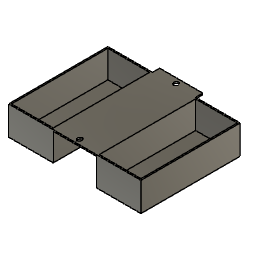
Load basket version 1 v3 (Autodesk Fusion 360 design; units mm, degrees)
Autodesk Fusion 360 part; units mm, degrees
note: some values were not read from the file. Set by a fixed rule: which face or edge a step refers to.
sketch "Sketch1" plane through (0, 0, 350) normal (0, 0, 1) x (-1, 0, 0)
  line L0 (-26.0008, 95.0009) -> (-26.0008, -144.9991)
  line L1 (-26.0008, -144.9991) -> (23.9992, -144.9991)
  line L2 (23.9992, -144.9991) -> (23.9992, 95.0009)
  line L3 (23.9992, 95.0009) -> (-26.0008, 95.0009)
  circle A0 centre (-0.9844, 75.5009) radius 10
  circle A1 centre (-1.0008, 8.5009) radius 10
  circle A2 centre (-1.0008, -58.4991) radius 10
  circle A3 centre (-0.9479, -125.4989) radius 10
  line L4 (5.9992, -44.9991) -> (5.9992, -4.9991)
  arc A4 (15.9992, -4.9991) -> (5.9992, -4.9991) centre (10.9992, -4.9991) ccw
  line L5 (15.9992, -4.9991) -> (15.9992, -44.9991)
  arc A5 (5.9992, -44.9991) -> (15.9992, -44.9991) centre (10.9992, -44.9991) ccw
  line L6 (-18.0008, 25.0009) -> (-18.0008, 60.0009)
  arc A6 (-8.0008, 60.0009) -> (-18.0008, 60.0009) centre (-13.0008, 60.0009) ccw
  line L7 (-8.0008, 60.0009) -> (-8.0008, 25.0009)
  arc A7 (-18.0008, 25.0009) -> (-8.0008, 25.0009) centre (-13.0008, 25.0009) ccw
  circle A8 centre (-0.9844, 42.0009) radius 4
  line L8 (-8.0008, -74.9991) -> (-8.0013, -109.9281)
  arc A9 (-18.0003, -109.9281) -> (-8.0013, -109.9281) centre (-13.0008, -109.9991) ccw
  line L9 (-18.0003, -109.9281) -> (-18.0008, -74.9991)
  arc A10 (-8.0008, -74.9991) -> (-18.0008, -74.9991) centre (-13.0008, -74.9991) ccw
  circle A11 centre (-0.9479, -91.9989) radius 4
  circle A12 centre (-1.0008, -24.9991) radius 4
  line L10 (-8.0008, -4.9991) -> (-8.0008, -44.9991)
  arc A13 (-18.0008, -44.9991) -> (-8.0008, -44.9991) centre (-13.0008, -44.9991) ccw
  line L11 (-18.0008, -44.9991) -> (-18.0008, -4.9991)
  arc A14 (-8.0008, -4.9991) -> (-18.0008, -4.9991) centre (-13.0008, -4.9991) ccw
  line L12 (5.9992, 25.0009) -> (5.9992, 60.0009)
  arc A15 (15.9992, 60.0009) -> (5.9992, 60.0009) centre (10.9992, 60.0009) ccw
  line L13 (15.9992, 60.0009) -> (15.9992, 25.0009)
  arc A16 (5.9992, 25.0009) -> (15.9992, 25.0009) centre (10.9992, 25.0009) ccw
  line L14 (5.9992, -109.9991) -> (5.9992, -74.9991)
  arc A17 (15.9992, -74.9991) -> (5.9992, -74.9991) centre (10.9992, -74.9991) ccw
  line L15 (15.9992, -74.9991) -> (15.9992, -109.9991)
  arc A18 (5.9992, -109.9991) -> (15.9992, -109.9991) centre (10.9992, -109.9991) ccw
  circle A19 centre (-0.9844, 42.0009) radius 4
  line L16 (26, 45) -> (26, 35)
  line L17 (26, 35) -> (-28, 35)
  line L18 (-28, 35) -> (-28, 45)
  line L19 (-28, 45) -> (-28, 49)
  line L20 (-28, 49) -> (26, 49)
  line L21 (26, 49) -> (26, 45)
  circle A20 centre (-0.9479, -91.9989) radius 4
  line L22 (-1, -85) -> (26, -85)
  line L23 (26, -85) -> (26, -98)
  line L24 (26, -98) -> (26, -99)
  line L25 (26, -99) -> (-28, -99)
  line L26 (-28, -99) -> (-28, -86)
  line L27 (-28, -86) -> (-28, -85)
  line L28 (-28, -85) -> (-1, -85)
  constraint concentric A8 A19
  constraint vertical L16
  constraint horizontal L17
  constraint vertical L18
  constraint vertical L19
  constraint horizontal L20
  constraint vertical L21
  constraint concentric A11 A20
  constraint perpendicular L2 L22
  constraint perpendicular L22 L23
  constraint parallel L2 L24
  constraint perpendicular L0 L25
  constraint perpendicular L25 L26
  constraint perpendicular L22 L27
  constraint parallel L22 L28
extrude "Extrude1" add sketch "Sketch1" along normal blind 2 contours L0 L9 L25 L28 | L0 L25 L26 L27 L28 | L8 L9 L25 L28 | L2 L22 L23 L24 L25 | L2 L15 L22 L25 | L8 L14 L22 L25 L28 | L14 L15 L22 L25 makes body 1
extrude "Extrude2" add sketch "Sketch1" along normal blind 2 separate body contours L0 L6 L17 L20 | L0 L17 L18 L19 L20 | L6 L7 L17 L20 | L2 L16 L17 L20 L21 | L2 L13 L17 L20 | L7 L12 L17 L20 | L12 L13 L17 L20 makes body 2
extrude "Extrude3" add 4 faces at (28, -46.3333, 350.6667) (28, -38.3333, 350.6667) (28, 85.6667, 350.6667) (28, 94.6667, 350.6667) along direction (1, 0, 0) blind 2 on bodies 1 2 bodies 2 1
sketch "Sketch3" plane through (30, 0, 0) normal (1, 0, 0) x (0, 1, 0)
  line L0 (-49, 350) -> (-35, 350)
  line L1 (-35, 350) -> (-35, 352)
  line L2 (-35, 352) -> (-49, 352)
  line L3 (-49, 352) -> (-49, 350)
  line L4 (-49, 352) -> (-35, 352)
  line L5 (-35, 352) -> (-35, 312)
  line L6 (-35, 312) -> (-49, 312)
  line L7 (-49, 312) -> (-49, 352)
  line L8 (85.0431, 352) -> (99, 352)
  line L9 (99, 352) -> (99, 312)
  line L10 (99, 312) -> (85.0431, 312)
  line L11 (85.0431, 352) -> (84.9998, 352)
  line L12 (84.9998, 352) -> (84.9998, 312)
  line L13 (84.9998, 312) -> (85.0431, 312)
  constraint horizontal L4
  constraint vertical L5
  constraint horizontal L6
  constraint vertical L7
  constraint coincident L2.end L3.start
  constraint horizontal L8
  constraint vertical L9
  constraint horizontal L10
  constraint horizontal L11
  constraint vertical L12
  constraint horizontal L13
extrude "Extrude4" add sketch "Sketch3" along normal blind 2 bodies 1 2
extrude "Extrude5" add 1 faces at (12, -35, 351.3333) along direction (0, 1, 0) blind 125 on bodies 2 bodies 2 1
extrude "Extrude6" cut sketch "Sketch1" along normal blind 15 contours A8 A19 | A11 A20 bodies 2
sketch "Sketch4" plane through (32, 0, 0) normal (1, 0, 0) x (0, 1, 0)
  line L0 (-49, 312) -> (99, 312)
  line L1 (99, 312) -> (99, 352)
  line L2 (99, 352) -> (-49, 352)
  line L3 (-49, 352) -> (-49, 312)
  line L4 (-49, 352) -> (-47, 352)
  line L5 (-47, 352) -> (-47, 312)
  line L6 (-47, 312) -> (-49, 312)
  line L7 (-49, 312) -> (-49, 352)
  line L8 (-47, 314) -> (99, 314)
  line L9 (99, 314) -> (99, 312)
  line L10 (99, 312) -> (-47, 312)
  line L11 (-47, 312) -> (-47, 314)
  line L12 (97, 314) -> (99, 314)
  line L13 (99, 314) -> (99, 352)
  line L14 (99, 352) -> (97, 352)
  line L15 (97, 352) -> (97, 314)
  constraint horizontal L4
  constraint vertical L5
  constraint horizontal L6
  constraint vertical L7
  constraint coincident L2.end L3.start
  constraint horizontal L8
  constraint vertical L9
  constraint horizontal L10
  constraint vertical L11
  constraint coincident L0.end L1.start
  constraint coincident L5 L8.start
  constraint horizontal L12
  constraint vertical L13
  constraint horizontal L14
  constraint vertical L15
  constraint coincident L1.end L2.start
  constraint coincident L8 L12.start
extrude "Extrude7" add sketch "Sketch4" along normal blind 30 contours L0 L2 L3 L4 L5 L6 L7 L11 | L0 L1 L5 L8 L9 L10 L11 L12 | L1 L2 L8 L12 L13 L14 L15 bodies 2
sketch "Sketch5" plane through (0, 0, 314) normal (0, 0, 1) x (-1, 0, 0)
  line L0 (-32, -97) -> (-32, 47)
  line L1 (-32, 47) -> (-62, 47)
  line L2 (-62, 47) -> (-62, -97)
  line L3 (-62, -97) -> (-32, -97)
  line L4 (-60, 47) -> (-62, 47)
  line L5 (-62, 47) -> (-62, -97)
  line L6 (-62, -97) -> (-60, -97)
  line L7 (-60, -97) -> (-60, 47)
  constraint horizontal L4
  constraint vertical L5
  constraint horizontal L6
  constraint vertical L7
  constraint coincident L2.end L3.start
  constraint coincident L1 L4.start
extrude "Extrude8" add sketch "Sketch5" along normal blind 38 contours L1 L2 L3 L4 L5 L6 L7 bodies 2
sketch "Sketch6" plane through (62, 0, 0) normal (1, 0, 0) x (0, 1, 0)
  line L0 (99, 312) -> (99, 352)
  line L1 (99, 352) -> (97, 352)
  line L2 (97, 352) -> (-47, 352)
  line L3 (-49, 352) -> (-49, 312)
  line L4 (-49, 312) -> (99, 312)
  line L5 (-47, 352) -> (99, 312) construction
  line L6 (99, 352) -> (-49, 312) construction
  line L7 (24, 347) -> (26, 347)
  line L8 (26, 347) -> (26, 317)
  line L9 (26, 317) -> (24, 317)
  line L10 (24, 317) -> (24, 347)
  line L11 (31, 347) -> (33, 347)
  line L12 (33, 347) -> (33, 317)
  line L13 (33, 317) -> (31, 317)
  line L14 (31, 317) -> (31, 347)
  line L15 (38, 347) -> (40, 347)
  line L16 (40, 347) -> (40, 317)
  line L17 (40, 317) -> (38, 317)
  line L18 (38, 317) -> (38, 347)
  line L19 (45, 317) -> (47, 317)
  line L20 (47, 317) -> (47, 347)
  line L21 (47, 347) -> (45, 347)
  line L22 (45, 347) -> (45, 317)
  line L23 (52, 347) -> (54, 347)
  line L24 (54, 347) -> (54, 317)
  line L25 (54, 317) -> (52, 317)
  line L26 (52, 317) -> (52, 347)
  line L27 (59, 317) -> (61, 317)
  line L28 (61, 317) -> (61, 347)
  line L29 (61, 347) -> (59, 347)
  line L30 (59, 347) -> (59, 317)
  line L31 (66, 347) -> (68, 347)
  line L32 (68, 347) -> (68, 317)
  line L33 (68, 317) -> (66, 317)
  line L34 (66, 317) -> (66, 347)
  line L35 (73, 317) -> (75, 317)
  line L36 (75, 317) -> (75, 347)
  line L37 (75, 347) -> (73, 347)
  line L38 (73, 347) -> (73, 317)
  line L39 (80, 347) -> (82, 347)
  line L40 (82, 347) -> (82, 317)
  line L41 (82, 317) -> (80, 317)
  line L42 (80, 317) -> (80, 347)
  line L43 (87, 347) -> (89, 347)
  line L44 (89, 347) -> (89, 317)
  line L45 (89, 317) -> (87, 317)
  line L46 (87, 317) -> (87, 347)
  line L47 (94, 347) -> (96, 347)
  line L48 (96, 347) -> (96, 317)
  line L49 (96, 317) -> (94, 317)
  line L50 (94, 317) -> (94, 347)
  line L51 (19, 347) -> (17, 347)
  line L52 (17, 347) -> (17, 317)
  line L53 (17, 317) -> (19, 317)
  line L54 (19, 317) -> (19, 347)
  line L55 (12, 347) -> (10, 347)
  line L56 (10, 347) -> (10, 317)
  line L57 (10, 317) -> (12, 317)
  line L58 (12, 317) -> (12, 347)
  line L59 (5, 317) -> (3, 317)
  line L60 (3, 317) -> (3, 347)
  line L61 (3, 347) -> (5, 347)
  line L62 (5, 347) -> (5, 317)
  line L63 (-2, 347) -> (-4, 347)
  line L64 (-4, 347) -> (-4, 317)
  line L65 (-4, 317) -> (-2, 317)
  line L66 (-2, 317) -> (-2, 347)
  line L67 (-9, 317) -> (-11, 317)
  line L68 (-11, 317) -> (-11, 347)
  line L69 (-11, 347) -> (-9, 347)
  line L70 (-9, 347) -> (-9, 317)
  line L71 (-16, 347) -> (-18, 347)
  line L72 (-18, 347) -> (-18, 317)
  line L73 (-18, 317) -> (-16, 317)
  line L74 (-16, 317) -> (-16, 347)
  line L75 (-23, 317) -> (-25, 317)
  line L76 (-25, 317) -> (-25, 347)
  line L77 (-25, 347) -> (-23, 347)
  line L78 (-23, 347) -> (-23, 317)
  line L79 (-30, 317) -> (-32, 317)
  line L80 (-32, 317) -> (-32, 347)
  line L81 (-32, 347) -> (-30, 347)
  line L82 (-30, 347) -> (-30, 317)
  line L83 (-37, 347) -> (-39, 347)
  line L84 (-39, 347) -> (-39, 317)
  line L85 (-39, 317) -> (-37, 317)
  line L86 (-37, 317) -> (-37, 347)
  line L87 (-44, 347) -> (-46, 347)
  line L88 (-46, 347) -> (-46, 317)
  line L89 (-46, 317) -> (-44, 317)
  line L90 (-44, 317) -> (-44, 347)
  line L91 (-47, 352) -> (-49, 352)
  constraint coincident L2.end L5.start
  constraint coincident L0.start L4.end
  constraint coincident L0.end L1.start
  constraint coincident L3.end L4.start
  constraint horizontal L7
  constraint vertical L8
  constraint horizontal L9
  constraint vertical L10
  constraint horizontal L11
  constraint vertical L12
  constraint horizontal L13
  constraint vertical L14
  constraint horizontal L15
  constraint vertical L16
  constraint horizontal L17
  constraint vertical L18
  constraint horizontal L19
  constraint vertical L20
  constraint horizontal L21
  constraint vertical L22
  constraint horizontal L23
  constraint vertical L24
  constraint horizontal L25
  constraint vertical L26
  constraint horizontal L27
  constraint vertical L28
  constraint horizontal L29
  constraint vertical L30
  constraint horizontal L31
  constraint vertical L32
  constraint horizontal L33
  constraint vertical L34
  constraint horizontal L35
  constraint vertical L36
  constraint horizontal L37
  constraint vertical L38
  constraint horizontal L39
  constraint vertical L40
  constraint horizontal L41
  constraint vertical L42
  constraint horizontal L43
  constraint vertical L44
  constraint horizontal L45
  constraint vertical L46
  constraint horizontal L47
  constraint vertical L48
  constraint horizontal L49
  constraint vertical L50
  constraint horizontal L51
  constraint vertical L52
  constraint horizontal L53
  constraint vertical L54
  constraint horizontal L55
  constraint vertical L56
  constraint horizontal L57
  constraint vertical L58
  constraint horizontal L59
  constraint vertical L60
  constraint horizontal L61
  constraint vertical L62
  constraint horizontal L63
  constraint vertical L64
  constraint horizontal L65
  constraint vertical L66
  constraint horizontal L67
  constraint vertical L68
  constraint horizontal L69
  constraint vertical L70
  constraint horizontal L71
  constraint vertical L72
  constraint horizontal L73
  constraint vertical L74
  constraint horizontal L75
  constraint vertical L76
  constraint horizontal L77
  constraint vertical L78
  constraint horizontal L79
  constraint vertical L80
  constraint horizontal L81
  constraint vertical L82
  constraint horizontal L83
  constraint vertical L84
  constraint horizontal L85
  constraint vertical L86
  constraint horizontal L87
  constraint vertical L88
  constraint horizontal L89
  constraint vertical L90
extrude "Extrude9" cut sketch "Sketch6" against normal blind 5 contours L7 L8 L9 L10 | L11 L12 L13 L14 | L15 L16 L17 L18 | L19 L20 L21 L22 | L23 L24 L25 L26 | L27 L28 L29 L30 | L31 L32 L33 L34 | L35 L36 L37 L38 | L39 L40 L41 L42 | L43 L44 L45 L46 | L47 L48 L49 L50 | L51 L52 L53 L54 | L55 L56 L57 L58 | L59 L60 L61 L62 | L63 L64 L65 L66 | L67 L68 L69 L70 | L71 L72 L73 L74 | L75 L76 L77 L78 | L79 L80 L81 L82 | L83 L84 L85 L86 | L87 L88 L89 L90 bodies 2
sketch "Sketch7" plane through (0, 0, 352) normal (0, 0, 1) x (-1, 0, 0)
  line L0 (-62, -97) -> (-62, -99)
  line L1 (-62, -99) -> (26, -99)
  line L2 (26, -99) -> (26, 49)
  line L3 (26, 49) -> (-62, 49)
  line L4 (-62, 49) -> (-62, 47)
  line L5 (-62, 47) -> (-62, -97)
  line L6 (-60, -97) -> (-60, 47)
  line L7 (-60, 47) -> (-32, 47)
  line L8 (-32, 47) -> (-32, -97)
  line L9 (-32, -97) -> (-60, -97)
  circle A0 centre (-0.9844, 42.0009) radius 4
  circle A1 centre (-0.9479, -91.9989) radius 4
  line L10 (-0.9844, 42.0009) -> (-0.9844, 49)
  line L11 (-0.9844, 42.0009) -> (-0.9844, -105)
  constraint coincident A0.centre L10.start
  constraint coincident L3 L10.end
  constraint perpendicular L3 L10
  constraint perpendicular L1 L11
mirror "Mirror1" about plane through (0, 0, 0) normal (1, 0, 0) of bodies 2 merged
extrude "Extrude10" add 1 faces at (-62, 24.6667, 350.3333) along direction (-1, 0, 0) blind 30 on bodies 2 bodies 2
extrude "Extrude11" add 1 faces at (62, 24.6667, 350.3333) along direction (1, 0, 0) blind 30 on bodies 2 bodies 2
extrude "Extrude12" cut 1 faces at (-60, 24.6667, 350.3333) along direction (-1, 0, 0) blind 30 on bodies 2 bodies 2
extrude "Extrude13" cut 1 faces at (60, 24.6667, 350.3333) along direction (1, 0, 0) blind 30 on bodies 2 bodies 2
sketch "Sketch8" plane through (0, -49, 0) normal (0, -1, 0) x (1, 0, 0)
  line L0 (-30, 350) -> (30, 350)
  line L1 (30, 350) -> (30, 312)
  line L2 (30, 312) -> (92, 312)
  line L3 (92, 312) -> (92, 352)
  line L4 (92, 352) -> (-92, 352)
  line L5 (-92, 352) -> (-92, 312)
  line L6 (-92, 312) -> (-30, 312)
  line L7 (-30, 312) -> (-30, 350)
  line L8 (-30, 312) -> (-92, 352) construction
  line L9 (-30, 352) -> (-92, 312) construction
  line L10 (-62, 317) -> (-60, 317)
  line L11 (-60, 317) -> (-60, 347)
  line L12 (-60, 347) -> (-62, 347)
  line L13 (-62, 347) -> (-62, 317)
  line L14 (-55, 347) -> (-53, 347)
  line L15 (-53, 347) -> (-53, 317)
  line L16 (-53, 317) -> (-55, 317)
  line L17 (-55, 317) -> (-55, 347)
  line L18 (-48, 347) -> (-46, 347)
  line L19 (-46, 347) -> (-46, 317)
  line L20 (-46, 317) -> (-48, 317)
  line L21 (-48, 317) -> (-48, 347)
  line L22 (-41, 347) -> (-39, 347)
  line L23 (-39, 347) -> (-39, 317)
  line L24 (-39, 317) -> (-41, 317)
  line L25 (-41, 317) -> (-41, 347)
  line L26 (-34, 347) -> (-32, 347)
  line L27 (-32, 347) -> (-32, 317)
  line L28 (-32, 317) -> (-34, 317)
  line L29 (-34, 317) -> (-34, 347)
  line L30 (-67, 347) -> (-69, 347)
  line L31 (-69, 347) -> (-69, 317)
  line L32 (-69, 317) -> (-67, 317)
  line L33 (-67, 317) -> (-67, 347)
  line L34 (-74, 317) -> (-76, 317)
  line L35 (-76, 317) -> (-76, 347)
  line L36 (-76, 347) -> (-74, 347)
  line L37 (-74, 347) -> (-74, 317)
  line L38 (-81, 347) -> (-83, 347)
  line L39 (-83, 347) -> (-83, 317)
  line L40 (-83, 317) -> (-81, 317)
  line L41 (-81, 317) -> (-81, 347)
  line L42 (-88, 317) -> (-90, 317)
  line L43 (-90, 317) -> (-90, 347)
  line L44 (-90, 347) -> (-88, 347)
  line L45 (-88, 347) -> (-88, 317)
  constraint coincident L6.end L7.start
  constraint coincident L4.end L5.start
  constraint coincident L4 L9.start
  constraint coincident L5.end L6.start
  constraint horizontal L10
  constraint vertical L11
  constraint horizontal L12
  constraint vertical L13
  constraint horizontal L14
  constraint vertical L15
  constraint horizontal L16
  constraint vertical L17
  constraint horizontal L18
  constraint vertical L19
  constraint horizontal L20
  constraint vertical L21
  constraint horizontal L22
  constraint vertical L23
  constraint horizontal L24
  constraint vertical L25
  constraint horizontal L26
  constraint vertical L27
  constraint horizontal L28
  constraint vertical L29
  constraint horizontal L30
  constraint vertical L31
  constraint horizontal L32
  constraint vertical L33
  constraint horizontal L34
  constraint vertical L35
  constraint horizontal L36
  constraint vertical L37
  constraint horizontal L38
  constraint vertical L39
  constraint horizontal L40
  constraint vertical L41
  constraint horizontal L42
  constraint vertical L43
  constraint horizontal L44
  constraint vertical L45
extrude "Extrude16" add 1 faces at (-91.3333, 96, 337) along direction (0, -1, 0) blind 145 on bodies 2 bodies 2
extrude "Extrude17" add 1 faces at (91.3333, 96, 337) along direction (0, -1, 0) blind 144 on bodies 2 bodies 2
sketch "Sketch11" plane through (0, 99, 0) normal (0, 1, 0) x (-1, 0, 0)
  line L0 (92, 352) -> (-92, 352)
  line L1 (-92, 352) -> (-92, 312)
  line L2 (-92, 312) -> (-30, 312)
  line L3 (-30, 312) -> (-30, 350)
  line L4 (-30, 350) -> (30, 350)
  line L5 (30, 350) -> (30, 312)
  line L6 (30, 312) -> (92, 312)
  line L7 (92, 312) -> (92, 352)
  line L8 (92, 352) -> (30, 352)
  line L9 (30, 352) -> (30, 312)
  line L10 (30, 312) -> (92, 312)
  line L11 (92, 312) -> (92, 352)
  line L12 (-30, 312) -> (-92, 312)
  line L13 (-92, 312) -> (-92, 352)
  line L14 (-92, 352) -> (-30, 352)
  line L15 (-30, 352) -> (-30, 312)
  constraint horizontal L8
  constraint vertical L9
  constraint horizontal L10
  constraint vertical L11
  constraint coincident L5.end L6.start
  constraint coincident L0.start L7.end
  constraint horizontal L12
  constraint vertical L13
  constraint horizontal L14
  constraint vertical L15
  constraint coincident L0.end L1.start
  constraint coincident L2.end L3.start
extrude "Extrude18" add 1 faces at (61.3333, 97, 326.6667) along direction (0, -1, 0) blind 10 on bodies 2 bodies 2
extrude "Extrude19" add 1 faces at (-61.3333, 97, 326.6667) along direction (0, -1, 0) blind 10 on bodies 2 bodies 2
extrude "Extrude20" cut sketch "Sketch11" against normal blind 10 contours L0 L5 L6 L7 L8 L9 L10 L11 | L0 L1 L2 L3 L12 L13 L14 L15 bodies 2
